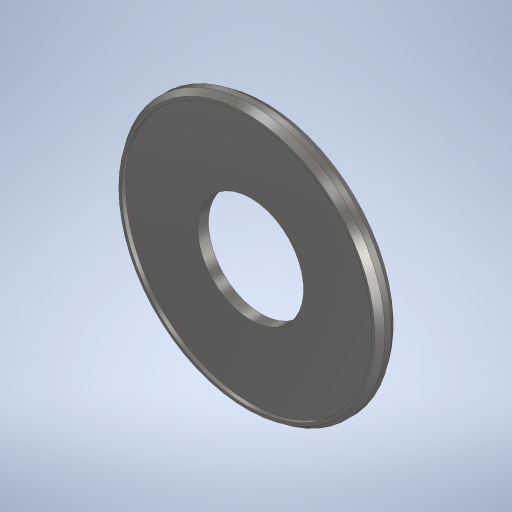
# Autodesk Inventor part: Clamex grooving Tool
Saved by Autodesk Inventor 2024 (Build 280153000, 153)
## iProperties
Created: 2021-09-07
Part Number: Clamex grooving Tool
Material: Stainless Steel
Document SubType Name: Modeling
Designer: sauliusd
Density: 8 g/cm^3
Appearance: Semi-Polished
Author: sauliusd
Autodesk Inventor part; units mm, degrees
ref_plane "YZ Plane" through (0, 0, 0) normal (1, 0, 0) x (0, 1, 0)
ref_plane "XZ Plane" through (0, 0, 0) normal (0, 1, 0) x (-1, 0, 0)
ref_plane "XY Plane" through (0, 0, 0) normal (0, 0, 1) x (1, 0, 0)
sketch "Sketch1" plane through (0, 0, 0) normal (1, 0, 0) x (0, 1, 0)
  circle A0 centre (0, 0) radius 50
  dimension "d0" = 100
  constraints: 1 centre point, 1 coincident
  measures "d0" diameter of A0
extrude "Extrusion1" add sketch "Sketch1" along normal mid plane 7
sketch "Sketch2" plane through (-3.5, 0, 0) normal (-1, 0, 0) x (0, 0, 1)
  circle A0 centre (0, 0) radius 50 projected
  circle A1 centre (0, 0) radius 47.3
  dimension "d4" = 47.3
  constraints: 1 centre point
  measures "d4" radius of A1
extrude "Extrusion2" cut sketch "Sketch2" against normal blind 1.5 contours A1
mirror "Mirror1" about plane through (0, 0, 0) normal (1, 0, 0) of "Extrusion2"
chamfer "Chamfer1" distance 1.61 angle 55 1 edges at (3.5, -50, 0) measured on face at (3.5, 0, -48.0382)
sketch "Sketch3" plane through (-2, 0, 0) normal (-1, 0, 0) x (0, 0, 1)
  circle A0 centre (0, 0) radius 20
  dimension "d10" = 40
  constraints: 1 centre point, 1 coincident
  measures "d10" diameter of A0
extrude "Extrusion3" cut sketch "Sketch3" against normal through all
chamfer "Chamfer2" distance 1.61 angle 55 1 edges at (-3.5, -50, 0) measured on face at (-3.5, 0, -48.0382)
equation "\"d13\" = d7"
equation "\"d7\" = 1.61"
body "Solid1"
